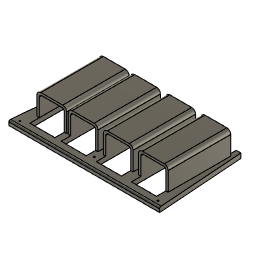
Actuator Securing Plate v1 v3 (Autodesk Fusion 360 design; units mm, degrees)
Autodesk Fusion 360 part; units mm, degrees
sketch "Sketch1" plane through (0, 0, 0) normal (0, 0, 1) x (1, 0, 0)
  line L0 (7.8365, 56.717) -> (95.1165, 56.717)
  line L1 (95.1165, 56.717) -> (99.132, 0.6987)
  line L2 (99.132, 0.6987) -> (2.632, 0.6987)
  line L3 (2.632, 0.6987) -> (7.8365, 56.717)
  dimension "d1" = 87.28
  dimension "d2" = 96.5
  dimension "d3" = 95.308
  dimension "d4" = 94.1
  constraint horizontal L0
  constraint parallel L0 L2
  measures "d1" distance of L0.start L0.end
  measures "d2" distance of L1.end L2.end
  measures "d3" angle of L0 L3
  measures "d4" angle of L0 L1
extrude "Extrude1" add sketch "Sketch1" along normal blind 3
sketch "Sketch2" plane through (0, 56.717, 0) normal (0, 1, 0) x (-1, 0, 0)
  line L0 (-95.1165, 0) -> (-7.8365, 0)
  line L1 (-7.8365, 0) -> (-7.8365, 3)
  line L2 (-7.8365, 3) -> (-95.1165, 3)
  line L3 (-95.1165, 3) -> (-95.1165, 0)
  line L4 (-92.1095, 3) -> (-92.1095, 16)
  line L5 (-92.1095, 16) -> (-76.1095, 16)
  line L6 (-76.1095, 16) -> (-76.1095, 3)
  line L7 (-69.6275, 3) -> (-69.6275, 16)
  line L8 (-69.6275, 16) -> (-53.6275, 16)
  line L9 (-53.6275, 16) -> (-53.6275, 3)
  line L10 (-47.1465, 3) -> (-47.1465, 16)
  line L11 (-47.1465, 16) -> (-31.1465, 16)
  line L12 (-31.1465, 16) -> (-31.1465, 3)
  line L13 (-27.0655, 3) -> (-27.0655, 16)
  line L14 (-27.0655, 16) -> (-11.0655, 16)
  line L15 (-11.0655, 16) -> (-11.0655, 3)
  line L16 (-74.6095, 17.5) -> (-74.6095, 3)
  line L17 (-71.1275, 3) -> (-71.1275, 17.5)
  line L18 (-48.6465, 3) -> (-48.6465, 17.5)
  line L19 (-48.6465, 17.5) -> (-29.6465, 17.5)
  line L20 (-29.6465, 17.5) -> (-29.6465, 3)
  line L21 (-28.5655, 3) -> (-28.5655, 17.5)
  line L22 (-28.5655, 17.5) -> (-9.5655, 17.5)
  line L23 (-9.5655, 17.5) -> (-9.5655, 3)
  line L24 (-74.6095, 17.5) -> (-93.6095, 17.5)
  line L25 (-93.6095, 17.5) -> (-93.6095, 3)
  line L26 (-71.1275, 17.5) -> (-52.1275, 17.5)
  line L27 (-52.1275, 17.5) -> (-52.1275, 3)
  dimension "d7" = 3.007
  dimension "d11" = 16
  dimension "d12" = 6.482
  dimension "d13" = 16
  dimension "d14" = 6.481
  dimension "d15" = 16
  dimension "d16" = 4.081
  dimension "d17" = 16
  dimension "d18" = 13
  dimension "d19" = 13
  dimension "d20" = 13
  dimension "d21" = 13
  dimension "d23" = 1.5
  dimension "d24" = 1.5
  dimension "d25" = 1.5
  dimension "d26" = 1.5
  dimension "d28" = 1.5
  dimension "d29" = 1.5
  dimension "d30" = 1.5
  dimension "d31" = 1.5
  dimension "d32" = 1.5
  dimension "d33" = 1.5
  dimension "d34" = 1.5
  dimension "d35" = 1.5
  constraint coincident L2 L4.start
  constraint perpendicular L2 L4
  constraint perpendicular L4 L5
  constraint coincident L2 L6.end
  constraint perpendicular L2 L6
  constraint coincident L2 L7.start
  constraint perpendicular L2 L7
  constraint perpendicular L6 L8
  constraint coincident L2 L9.end
  constraint perpendicular L2 L9
  constraint coincident L2 L10.start
  constraint perpendicular L2 L10
  constraint perpendicular L10 L11
  constraint coincident L2 L12.end
  constraint perpendicular L2 L12
  constraint coincident L2 L13.start
  constraint perpendicular L2 L13
  constraint perpendicular L10 L14
  constraint coincident L2 L15.end
  constraint perpendicular L2 L15
  constraint coincident L2 L16.end
  constraint perpendicular L2 L16
  constraint coincident L2 L17.start
  constraint perpendicular L2 L17
  constraint coincident L2 L18.start
  constraint perpendicular L2 L18
  constraint perpendicular L18 L19
  constraint coincident L2 L20.end
  constraint perpendicular L2 L20
  constraint coincident L2 L21.start
  constraint perpendicular L14 L21
  constraint perpendicular L21 L22
  constraint coincident L2 L23.end
  constraint perpendicular L2 L23
  constraint perpendicular L4 L24
  constraint coincident L2 L25.end
  constraint perpendicular L2 L25
  constraint perpendicular L17 L26
  constraint coincident L2 L27.end
  constraint perpendicular L2 L27
  measures "d7" distance of L2.end L4.start
  measures "d11" distance of L4.end L5.end
  measures "d12" distance of L6.end L7.start
  measures "d13" distance of L7.end L8.end
  measures "d14" distance of L9.end L10.start
  measures "d15" distance of L10.end L11.end
  measures "d16" distance of L12.end L13.start
  measures "d17" distance of L13.end L14.end
  measures "d18" distance of L4.start L4.end
  measures "d19" distance of L7.start L7.end
  measures "d20" distance of L10.start L10.end
  measures "d21" distance of L13.start L13.end
  measures "d23" distance of L4 L25
  measures "d24" distance of L5 L24
  measures "d25" distance of L6 L16
  measures "d26" distance of L7 L17
  measures "d28" distance of L10 L18
  measures "d29" distance of L11 L19
  measures "d30" distance of L12 L20
  measures "d31" distance of L13 L21
  measures "d32" distance of L14 L22
  measures "d33" distance of L15 L23
  measures "d34" distance of L9 L27
  measures "d35" distance of L8 L26
extrude "Extrude2" add sketch "Sketch2" against normal blind 40 from surface at -5 contours L2 L4 L5 L6 L16 L24 L25 | L2 L13 L14 L15 L21 L22 L23 | L2 L7 L8 L9 L17 L26 L27 | L2 L10 L11 L12 L18 L19 L20
sketch "Sketch3" plane through (0, 56.717, 0) normal (0, 1, 0) x (-1, 0, 0)
  line L0 (-95.1165, 0) -> (-7.8365, 0)
  line L1 (-7.8365, 0) -> (-7.8365, 3)
  line L2 (-7.8365, 3) -> (-95.1165, 3)
  line L3 (-95.1165, 3) -> (-95.1165, 0)
  line L4 (-92.1095, 3) -> (-76.1095, 3)
  line L5 (-76.1095, 0) -> (-92.1095, 0)
  line L6 (-92.1095, 3) -> (-92.1095, 0)
  line L7 (-76.1095, 3) -> (-76.1095, 0)
  line L8 (-69.6275, 3) -> (-69.6275, 0)
  line L9 (-69.6275, 3) -> (-53.6275, 3)
  line L10 (-53.6275, 0) -> (-53.6275, 3)
  line L11 (-53.6275, 0) -> (-69.6275, 0)
  line L12 (-47.1465, 3) -> (-47.1465, 0)
  line L13 (-47.1465, 3) -> (-31.1465, 3)
  line L14 (-31.1465, 0) -> (-31.1465, 3)
  line L15 (-31.1465, 0) -> (-47.1465, 0)
  line L16 (-27.0925, 3) -> (-11.0925, 3)
  line L17 (-11.0925, 0) -> (-11.0925, 3)
  line L18 (-11.0925, 0) -> (-27.0925, 0)
  line L19 (-27.0925, 3) -> (-27.0925, 0)
  dimension "d39" = 16
  dimension "d40" = 16
  dimension "d41" = 16
  dimension "d42" = 16
  dimension "d43" = 3.007
  dimension "d44" = 6.482
  dimension "d45" = 6.481
  dimension "d46" = 4.054
  constraint coincident L2 L4.start
  constraint coincident L2 L4.end
  constraint coincident L0 L5.start
  constraint coincident L0 L5.end
  constraint parallel L0 L5
  constraint perpendicular L5 L7
  constraint coincident L2 L8.start
  constraint coincident L0 L8.end
  constraint perpendicular L0 L8
  constraint coincident L2 L9.end
  constraint coincident L0 L10.start
  constraint perpendicular L9 L10
  constraint coincident L2 L12.start
  constraint coincident L0 L12.end
  constraint perpendicular L0 L12
  constraint coincident L2 L13.end
  constraint coincident L0 L14.start
  constraint perpendicular L13 L14
  constraint coincident L2 L16.start
  constraint coincident L2 L16.end
  constraint coincident L0 L17.start
  constraint perpendicular L16 L17
  constraint coincident L0 L18.end
  constraint perpendicular L17 L18
  constraint perpendicular L16 L19
  constraint parallel L6 L7
  measures "d39" distance of L6 L7
  measures "d40" distance of L8 L10
  measures "d41" distance of L12 L14
  measures "d42" distance of L17 L19
  measures "d43" distance of L3 L6
  measures "d44" distance of L7 L8
  measures "d45" distance of L10 L12
  measures "d46" distance of L14 L19
extrude "Extrude3" cut sketch "Sketch3" against normal blind 51 contours L0 L2 L4 L5 L6 L7 | L0 L2 L8 L9 L10 L11 | L0 L2 L12 L13 L14 L15 | L0 L2 L16 L17 L18 L19
fillet "Fillet1" radius 2.5 1 edges at (93.6095, 31.717, 17.5)
fillet "Fillet2" radius 2.5 7 edges at (74.6095, 31.717, 17.5) (71.1275, 31.717, 17.5) (52.1275, 31.717, 17.5) (48.6465, 31.717, 17.5) (29.6465, 31.717, 17.5) (9.5655, 31.717, 17.5) (28.5655, 31.717, 17.5)
fillet "Fillet3" radius 1 1 edges at (50.882, 0.6987, 3)
fillet "Fillet4" radius 1.5 2 edges at (27.0655, 31.717, 16) (11.0655, 31.717, 16)
fillet "Fillet4" radius 1.5 6 edges at (31.1465, 31.717, 16) (53.6275, 31.717, 16) (76.1095, 31.717, 16) (47.1465, 31.717, 16) (69.6275, 31.717, 16) (92.1095, 31.717, 16)
sketch "Sketch4" plane through (0, 0, 3) normal (0, 0, 1) x (-1, 0, 0)
  line L0 (-9.5655, -11.717) -> (-9.5655, -51.717)
  line L1 (-9.5655, -51.717) -> (-11.0655, -51.717)
  line L2 (-11.0655, -51.717) -> (-11.0655, -11.717)
  line L3 (-11.0655, -11.717) -> (-9.5655, -11.717)
  line L4 (-2.7249, -1.6987) -> (-99.0603, -1.6987)
  line L5 (-99.0603, -1.6987) -> (-95.1165, -56.717)
  line L6 (-95.1165, -56.717) -> (-92.1095, -56.717)
  line L7 (-92.1095, -56.717) -> (-92.1095, -51.717)
  line L8 (-92.1095, -51.717) -> (-93.6095, -51.717)
  line L9 (-93.6095, -51.717) -> (-93.6095, -11.717)
  line L10 (-93.6095, -11.717) -> (-92.1095, -11.717)
  line L11 (-92.1095, -11.717) -> (-92.1095, -5.717)
  line L12 (-92.1095, -5.717) -> (-76.1095, -5.717)
  line L13 (-76.1095, -5.717) -> (-76.1095, -11.717)
  line L14 (-76.1095, -11.717) -> (-74.6095, -11.717)
  line L15 (-74.6095, -11.717) -> (-74.6095, -51.717)
  line L16 (-74.6095, -51.717) -> (-76.1095, -51.717)
  line L17 (-76.1095, -51.717) -> (-76.1095, -56.717)
  line L18 (-76.1095, -56.717) -> (-69.6275, -56.717)
  line L19 (-69.6275, -56.717) -> (-69.6275, -51.717)
  line L20 (-69.6275, -51.717) -> (-71.1275, -51.717)
  line L21 (-71.1275, -51.717) -> (-71.1275, -11.717)
  line L22 (-71.1275, -11.717) -> (-69.6275, -11.717)
  line L23 (-69.6275, -11.717) -> (-69.6275, -5.717)
  line L24 (-69.6275, -5.717) -> (-53.6275, -5.717)
  line L25 (-53.6275, -5.717) -> (-53.6275, -11.717)
  line L26 (-53.6275, -11.717) -> (-52.1275, -11.717)
  line L27 (-52.1275, -11.717) -> (-52.1275, -51.717)
  line L28 (-52.1275, -51.717) -> (-53.6275, -51.717)
  line L29 (-53.6275, -51.717) -> (-53.6275, -56.717)
  line L30 (-53.6275, -56.717) -> (-47.1465, -56.717)
  line L31 (-47.1465, -56.717) -> (-47.1465, -51.717)
  line L32 (-47.1465, -51.717) -> (-48.6465, -51.717)
  line L33 (-48.6465, -51.717) -> (-48.6465, -11.717)
  line L34 (-48.6465, -11.717) -> (-47.1465, -11.717)
  line L35 (-47.1465, -11.717) -> (-47.1465, -5.717)
  line L36 (-47.1465, -5.717) -> (-31.1465, -5.717)
  line L37 (-31.1465, -5.717) -> (-31.1465, -11.717)
  line L38 (-31.1465, -11.717) -> (-29.6465, -11.717)
  line L39 (-29.6465, -11.717) -> (-29.6465, -51.717)
  line L40 (-29.6465, -51.717) -> (-31.1465, -51.717)
  line L41 (-31.1465, -51.717) -> (-31.1465, -56.717)
  line L42 (-31.1465, -56.717) -> (-27.0925, -56.717)
  line L43 (-27.0925, -56.717) -> (-27.0925, -51.717)
  line L44 (-27.0925, -51.717) -> (-28.5655, -51.717)
  line L45 (-28.5655, -51.717) -> (-28.5655, -11.717)
  line L46 (-28.5655, -11.717) -> (-27.0925, -11.717)
  line L47 (-27.0925, -11.717) -> (-27.0925, -5.717)
  line L48 (-27.0925, -5.717) -> (-11.0925, -5.717)
  line L49 (-11.0925, -5.717) -> (-11.0925, -56.717)
  line L50 (-11.0925, -56.717) -> (-7.8365, -56.717)
  line L51 (-7.8365, -56.717) -> (-2.7249, -1.6987)
  circle A0 centre (-50.1165, -53.717) radius 0.6186
  circle A1 centre (-6.7249, -3.717) radius 0.5
  circle A2 centre (-95.0603, -3.717) radius 0.5
  circle A3 centre (-50.3865, -7.717) radius 0.5
  dimension "d59" = 3
  dimension "d60" = 3.511
  dimension "d61" = 1
  dimension "d63" = 2
  dimension "d64" = 4
  dimension "d65" = 1
  dimension "d66" = 4
  dimension "d67" = 2
  dimension "d68" = 1
  dimension "d69" = 3.24
  dimension "d70" = 2
  measures "d59" distance of L30 A0.centre
  measures "d60" distance of L29 A0.centre
  measures "d61" diameter of A1
  measures "d63" distance of L48 A1.centre
  measures "d64" horizontal distance of L4.start A1.centre
  measures "d65" diameter of A2
  measures "d66" horizontal distance of L4.end A2.centre
  measures "d67" distance of L12 A2.centre
  measures "d68" diameter of A3
  measures "d69" distance of L35 A3.centre
  measures "d70" distance of L24 A3.centre
hole "Hole1" at (50.1165, 53.717, 3) at (6.7249, 3.717, 3) at (50.3865, 7.717, 3) at (95.0603, 3.717, 3) direction (0, 0, -1) diameter 1 depth 1.5 tip angle 118
